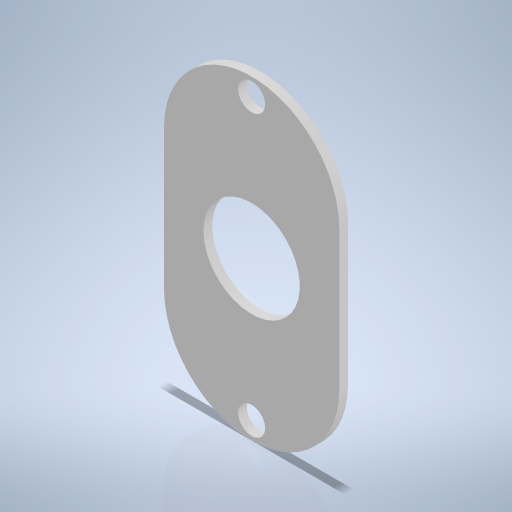
# Autodesk Inventor part: Deckscheibe
Saved by Autodesk Inventor 2024 (Build 280153000, 153)
## iProperties
Created: 2024-04-30
Part Number: Deckscheibe
Material: Generisch
Document SubType Name: Modeling
Designer: ffogue
Density: 1 g/cm^3
Appearance: Vorgabe
Author: ffogue
Autodesk Inventor part; units mm, degrees
ref_plane "YZ Plane" through (0, 0, 0) normal (1, 0, 0) x (0, 1, 0)
ref_plane "XZ Plane" through (0, 0, 0) normal (0, 1, 0) x (-1, 0, 0)
ref_plane "XY Plane" through (0, 0, 0) normal (0, 0, 1) x (1, 0, 0)
sketch "Skizze1" plane through (0, 0, 0) normal (0, 1, 0) x (-1, 0, 0)
  line L0 (0, 8) -> (0, -8) construction
  line L1 (-10, 8) -> (-10, -8)
  line L2 (10, -8) -> (10, 8)
  arc A0 (10, 8) -> (-10, 8) centre (0, 8) ccw
  arc A1 (-10, -8) -> (10, -8) centre (0, -8) ccw
  point P0 (0, 0)
  point P1 (0, 0)
  dimension "d0" = 10
  dimension "d1" = 16
  constraints: 8 end point, 4 point on circle, 4 tangent, 2 centre point, 1 coincident, 1 midpoint, 1 parallel, 1 vertical
  measures "d0" radius of A1
  measures "d1" distance of L0.start L0.end
extrude "Extrusion1" add sketch "Skizze1" along normal blind 1
sketch "Skizze2" plane through (0, 1, 0) normal (0, 1, 0) x (1, 0, 0)
  point P0 (0, 0)
  point P1 (0, -16)
  point P2 (0, 16)
  dimension "d11" = 32
  dimension "d12" = 16
  constraints: 2 vertical alignment
  measures "d11" distance of point (0, 16) point (0, -16)
  measures "d12" distance of point (0, 0) point (0, -16)
hole "Bohrung1" at (0, 1, 16) at (0, 1, -16) direction (0, -1, 0) diameter 3.1 depth 1
hole "Bohrung2" at (0, 1, 0) direction (0, -1, 0) diameter 11 depth 1
